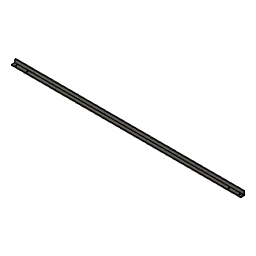
L channel 25x25x3 v2 (Autodesk Fusion 360 design; units mm, degrees)
Autodesk Fusion 360 part; units mm, degrees
sketch "Sketch1" plane through (0, 0, 0) normal (1, 0, 0) x (0, 1, 0)
  line L0 (-12.5, 0) -> (12.5, 0)
  line L1 (12.5, 0) -> (12.5, 25)
  line L2 (12.5, 25) -> (9.5, 25)
  line L3 (9.5, 25) -> (9.5, 3)
  line L4 (9.5, 3) -> (-12.5, 3)
  line L5 (-12.5, 3) -> (-12.5, 0)
  dimension "d2" = 25
  dimension "d3" = 25
  dimension "d4" = 3
  dimension "d5" = 22
  dimension "d6" = 22
  constraint perpendicular L1 L2
  constraint perpendicular L1 L4
  measures "d2" distance of L0.start L0.end
  measures "d3" distance of L0.end L1.end
  measures "d4" distance of L1.end L2.end
  measures "d5" distance of L2.end L3.end
  measures "d6" distance of L3.end L4.end
extrude "Extrude1" add sketch "Sketch1" along normal mid plane 1500
sketch "Sketch2" plane through (0, 0, 0) normal (0, 0, -1) x (1, 0, 0)
  line L0 (-750, -12.5) -> (750, -12.5)
  line L1 (750, -12.5) -> (750, 12.5)
  line L2 (750, 12.5) -> (-750, 12.5)
  line L3 (-750, 12.5) -> (-750, -12.5)
  line L4 (-750, 0) -> (-730, 0) construction
  line L5 (-730, 0) -> (-660, 0) construction
  line L6 (750, 0) -> (730, 0) construction
  line L7 (730, 0) -> (660, 0) construction
  dimension "d9" = 20
  dimension "d10" = 70
  dimension "d11" = 20
  dimension "d12" = 70
  constraint midpoint L3 L4.start
  constraint perpendicular L3 L4
  constraint perpendicular L3 L5
  constraint midpoint L1 L6.start
  constraint perpendicular L1 L6
  constraint perpendicular L1 L7
  measures "d9" distance of L4.start L4.end
  measures "d10" distance of L4.end L5.end
  measures "d11" distance of L6.start L6.end
  measures "d12" distance of L6.end L7.end
hole "Hole1" at (-660, 0, 0) at (-730, 0, 0) at (730, 0, 0) at (660, 0, 0) direction (0, 0, 1) diameter 5.5 depth 3 tip angle 180
